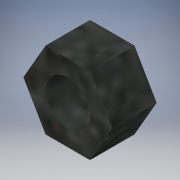
# Autodesk Inventor part: Parts_Nuts_M4
Saved by Autodesk Inventor 2019.1 (Build 231200000, 200)
## iProperties
Created: 2018-08-27
Part Number: Parts_Nuts_M4
Material: 鋼
Document SubType Name: Modeling
Designer: sktom
Density: 7.85 g/cm^3
Appearance: プレート
Author: sktom
Autodesk Inventor part; units mm, degrees
ref_plane "YZ Plane" through (0, 0, 0) normal (1, 0, 0) x (0, 1, 0)
ref_plane "XZ Plane" through (0, 0, 0) normal (0, 1, 0) x (-1, 0, 0)
ref_plane "XY Plane" through (0, 0, 0) normal (0, 0, 1) x (1, 0, 0)
sketch "スケッチ1" plane through (0, 0, 0) normal (0, 0, 1) x (1, 0, 0)
  line L0 (4, 0) -> (2, -3.4641)
  line L1 (2, -3.4641) -> (-2, -3.4641)
  line L2 (-2, -3.4641) -> (-4, 0)
  line L3 (-4, 0) -> (-2, 3.4641)
  line L4 (-2, 3.4641) -> (2, 3.4641)
  line L5 (2, 3.4641) -> (4, 0)
  circle A0 centre (0, 0) radius 2
  dimension "d0" = 8
  dimension "d1" = 4
  constraints: 12 end point, 2 coincident, 1 centre point, 1 horizontal, 13 other
  measures "d0" distance of L2.end L0.start
  measures "d1" diameter of A0
extrude "押し出し1" add sketch "スケッチ1" along normal blind 4
